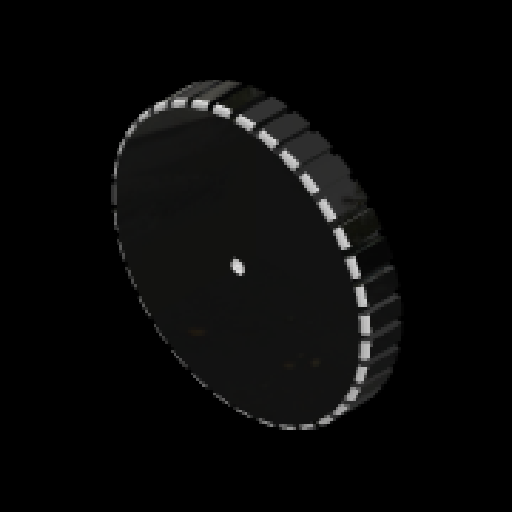
# Autodesk Inventor part: RobotWheelMK1
Saved by Autodesk Inventor 2025 (Build 290162000, 162)
## iProperties
Created: 2024-11-18
Part Number: RobotWheelMK1
Material: Generic
Document SubType Name: Modeling
Designer: Trevor
Density: 1 g/cm^3
Appearance: Default
Author: Trevor
Autodesk Inventor part; units mm, degrees
ref_plane "YZ Plane" through (0, 0, 0) normal (1, 0, 0) x (0, 1, 0)
ref_plane "XZ Plane" through (0, 0, 0) normal (0, 1, 0) x (-1, 0, 0)
sketch "Sketch1" plane through (0, 0, 0) normal (0, 0, 1) x (1, 0, 0)
  line L0 (-2.4408, -0.5408) -> (-1.2026, 2.1918) projected
  arc A0 (-2.4408, -0.5408) -> (-1.2026, 2.1918) centre (0, 0) ccw projected
  circle A1 centre (0, 0) radius 50
  line L1 (-52.2966, -3.2808) -> (-49.8922, -3.2808)
  line L2 (-49.8922, 3.2808) -> (-52.2966, 3.2808)
  line L3 (-52.2966, 3.2808) -> (-52.2966, -3.2808)
  line L4 (-52.2966, -3.2808) -> (-50, 0) construction
  line L5 (-50, 0) -> (-52.2966, 3.2808) construction
  line L6 (-49.6763, -5.6805) -> (-52.042, -6.1098)
  line L7 (-52.042, -6.1098) -> (-50.8703, -12.566)
  line L8 (-50.8703, -12.566) -> (-48.5046, -12.1367)
  circle A2 centre (0, 0) radius 50
  line L9 (-47.8637, -14.4592) -> (-50.1147, -15.3041)
  line L10 (-50.1147, -15.3041) -> (-47.8091, -21.4473)
  line L11 (-47.8091, -21.4473) -> (-45.5581, -20.6025)
  circle A3 centre (0, 0) radius 50
  line L12 (-44.5127, -22.7733) -> (-46.5767, -24.0064)
  line L13 (-46.5767, -24.0064) -> (-43.2112, -29.6393)
  line L14 (-43.2112, -29.6393) -> (-41.1472, -28.4061)
  circle A4 centre (0, 0) radius 50
  line L15 (-39.731, -30.3553) -> (-41.5417, -31.9372)
  line L16 (-41.5417, -31.9372) -> (-37.2245, -36.8787)
  line L17 (-37.2245, -36.8787) -> (-35.4138, -35.2967)
  circle A5 centre (0, 0) radius 50
  line L18 (-33.6724, -36.9618) -> (-35.1715, -38.8415)
  line L19 (-35.1715, -38.8415) -> (-30.0413, -42.9327)
  line L20 (-30.0413, -42.9327) -> (-28.5422, -41.0529)
  circle A6 centre (0, 0) radius 50
  line L21 (-26.5315, -42.3802) -> (-27.6708, -44.4975)
  line L22 (-27.6708, -44.4975) -> (-21.8926, -47.6068)
  line L23 (-21.8926, -47.6068) -> (-20.7533, -45.4896)
  circle A7 centre (0, 0) radius 50
  line L24 (-18.5378, -46.4365) -> (-19.2808, -48.7232)
  line L25 (-19.2808, -48.7232) -> (-13.0403, -50.7508)
  line L26 (-13.0403, -50.7508) -> (-12.2973, -48.4642)
  circle A8 centre (0, 0) radius 50
  line L27 (-9.9483, -49.0003) -> (-10.2711, -51.3829)
  line L28 (-10.2711, -51.3829) -> (-3.7688, -52.2637)
  line L29 (-3.7688, -52.2637) -> (-3.4461, -49.8811)
  circle A9 centre (0, 0) radius 50
  line L30 (-1.0391, -49.9892) -> (-0.9313, -52.3911)
  line L31 (-0.9313, -52.3911) -> (5.6238, -52.0967)
  line L32 (5.6238, -52.0967) -> (5.5159, -49.6948)
  circle A10 centre (0, 0) radius 50
  line L33 (7.9035, -49.3714) -> (8.4385, -51.7155)
  line L34 (8.4385, -51.7155) -> (14.8357, -50.2553)
  line L35 (14.8357, -50.2553) -> (14.3007, -47.9113)
  circle A11 centre (0, 0) radius 50
  line L36 (16.5921, -47.1668) -> (17.537, -49.3776)
  line L37 (17.537, -49.3776) -> (23.5707, -46.7987)
  line L38 (23.5707, -46.7987) -> (22.6257, -44.5879)
  circle A12 centre (0, 0) radius 50
  line L39 (24.7474, -43.4461) -> (26.0719, -45.4527)
  line L40 (26.0719, -45.4527) -> (31.5481, -41.8379)
  line L41 (31.5481, -41.8379) -> (30.2236, -39.8313)
  circle A13 centre (0, 0) radius 50
  line L42 (32.1073, -38.3291) -> (33.7688, -40.067)
  line L43 (33.7688, -40.067) -> (38.5116, -35.5324)
  line L44 (38.5116, -35.5324) -> (36.85, -33.7946)
  circle A14 centre (0, 0) radius 50
  line L45 (38.4352, -31.9802) -> (40.3804, -33.3934)
  line L46 (40.3804, -33.3934) -> (44.2373, -28.0849)
  line L47 (44.2373, -28.0849) -> (42.2921, -26.6717)
  circle A15 centre (0, 0) radius 50
  line L48 (43.5279, -24.6034) -> (45.6941, -25.6466)
  line L49 (45.6941, -25.6466) -> (48.5411, -19.7347)
  line L50 (48.5411, -19.7347) -> (46.3749, -18.6915)
  circle A16 centre (0, 0) radius 50
  line L51 (47.2214, -16.4358) -> (49.5391, -17.0754)
  line L52 (49.5391, -17.0754) -> (51.2848, -10.7502)
  line L53 (51.2848, -10.7502) -> (48.9671, -10.1106)
  circle A17 centre (0, 0) radius 50
  line L54 (49.3973, -7.7399) -> (51.792, -7.9555)
  line L55 (51.792, -7.9555) -> (52.3801, -1.4202)
  line L56 (52.3801, -1.4202) -> (49.9855, -1.2047)
  circle A18 centre (0, 0) radius 50
  line L57 (49.9855, 1.2047) -> (52.3801, 1.4202)
  line L58 (52.3801, 1.4202) -> (51.792, 7.9555)
  line L59 (51.792, 7.9555) -> (49.3973, 7.7399)
  circle A19 centre (0, 0) radius 50
  line L60 (48.9671, 10.1106) -> (51.2848, 10.7502)
  line L61 (51.2848, 10.7502) -> (49.5391, 17.0754)
  line L62 (49.5391, 17.0754) -> (47.2214, 16.4358)
  circle A20 centre (0, 0) radius 50
  line L63 (46.3749, 18.6915) -> (48.5411, 19.7347)
  line L64 (48.5411, 19.7347) -> (45.6941, 25.6466)
  line L65 (45.6941, 25.6466) -> (43.5279, 24.6034)
  circle A21 centre (0, 0) radius 50
  line L66 (42.2921, 26.6717) -> (44.2373, 28.0849)
  line L67 (44.2373, 28.0849) -> (40.3804, 33.3934)
  line L68 (40.3804, 33.3934) -> (38.4352, 31.9802)
  circle A22 centre (0, 0) radius 50
  line L69 (36.85, 33.7946) -> (38.5116, 35.5324)
  line L70 (38.5116, 35.5324) -> (33.7688, 40.067)
  line L71 (33.7688, 40.067) -> (32.1073, 38.3291)
  circle A23 centre (0, 0) radius 50
  line L72 (30.2236, 39.8313) -> (31.5481, 41.8379)
  line L73 (31.5481, 41.8379) -> (26.0719, 45.4527)
  line L74 (26.0719, 45.4527) -> (24.7474, 43.4461)
  circle A24 centre (0, 0) radius 50
  line L75 (22.6257, 44.5879) -> (23.5707, 46.7987)
  line L76 (23.5707, 46.7987) -> (17.537, 49.3776)
  line L77 (17.537, 49.3776) -> (16.5921, 47.1668)
  circle A25 centre (0, 0) radius 50
  line L78 (14.3007, 47.9113) -> (14.8357, 50.2553)
  line L79 (14.8357, 50.2553) -> (8.4385, 51.7155)
  line L80 (8.4385, 51.7155) -> (7.9035, 49.3714)
  circle A26 centre (0, 0) radius 50
  line L81 (5.5159, 49.6948) -> (5.6238, 52.0967)
  line L82 (5.6238, 52.0967) -> (-0.9313, 52.3911)
  line L83 (-0.9313, 52.3911) -> (-1.0391, 49.9892)
  circle A27 centre (0, 0) radius 50
  line L84 (-3.4461, 49.8811) -> (-3.7688, 52.2637)
  line L85 (-3.7688, 52.2637) -> (-10.2711, 51.3829)
  line L86 (-10.2711, 51.3829) -> (-9.9483, 49.0003)
  circle A28 centre (0, 0) radius 50
  line L87 (-12.2973, 48.4642) -> (-13.0403, 50.7508)
  line L88 (-13.0403, 50.7508) -> (-19.2808, 48.7232)
  line L89 (-19.2808, 48.7232) -> (-18.5378, 46.4365)
  circle A29 centre (0, 0) radius 50
  line L90 (-20.7533, 45.4896) -> (-21.8926, 47.6068)
  line L91 (-21.8926, 47.6068) -> (-27.6708, 44.4975)
  line L92 (-27.6708, 44.4975) -> (-26.5315, 42.3802)
  circle A30 centre (0, 0) radius 50
  line L93 (-28.5422, 41.0529) -> (-30.0413, 42.9327)
  line L94 (-30.0413, 42.9327) -> (-35.1715, 38.8415)
  line L95 (-35.1715, 38.8415) -> (-33.6724, 36.9618)
  circle A31 centre (0, 0) radius 50
  line L96 (-35.4138, 35.2967) -> (-37.2245, 36.8787)
  line L97 (-37.2245, 36.8787) -> (-41.5417, 31.9372)
  line L98 (-41.5417, 31.9372) -> (-39.731, 30.3553)
  circle A32 centre (0, 0) radius 50
  line L99 (-41.1472, 28.4061) -> (-43.2112, 29.6393)
  line L100 (-43.2112, 29.6393) -> (-46.5767, 24.0064)
  line L101 (-46.5767, 24.0064) -> (-44.5127, 22.7733)
  circle A33 centre (0, 0) radius 50
  line L102 (-45.5581, 20.6025) -> (-47.8091, 21.4473)
  line L103 (-47.8091, 21.4473) -> (-50.1147, 15.3041)
  line L104 (-50.1147, 15.3041) -> (-47.8637, 14.4592)
  circle A34 centre (0, 0) radius 50
  line L105 (-48.5046, 12.1367) -> (-50.8703, 12.566)
  line L106 (-50.8703, 12.566) -> (-52.042, 6.1098)
  line L107 (-52.042, 6.1098) -> (-49.6763, 5.6805)
  circle A35 centre (0, 0) radius 50
  line L108 (-1.3578, 2.3337) -> (-2.6499, -0.5177)
  arc A36 (-2.6499, -0.5177) -> (-1.3578, 2.3337) centre (0, 0) ccw
  point P0 (0, 0)
  point P1 (-49.1965, -8.9278)
  point P2 (-46.8117, -17.5687)
  point P3 (-42.9224, -25.645)
  point P4 (-37.6536, -32.8969)
  point P5 (-31.1745, -39.0916)
  point P6 (-23.6934, -44.0298)
  point P7 (-15.4508, -47.5528)
  point P8 (-6.7117, -49.5475)
  point P9 (2.2432, -49.9497)
  point P10 (11.126, -48.7464)
  point P11 (19.6513, -45.9764)
  point P12 (27.5448, -41.7287)
  point P13 (34.5531, -36.1397)
  point P14 (40.4508, -29.3893)
  point P15 (45.0484, -21.6942)
  point P16 (48.1981, -13.3018)
  point P17 (49.7987, -4.482)
  point P18 (49.7987, 4.482)
  point P19 (48.1981, 13.3018)
  point P20 (45.0484, 21.6942)
  point P21 (40.4508, 29.3893)
  point P22 (34.5531, 36.1397)
  point P23 (27.5448, 41.7287)
  point P24 (19.6513, 45.9764)
  point P25 (11.126, 48.7464)
  point P26 (2.2432, 49.9497)
  point P27 (-6.7117, 49.5475)
  point P28 (-15.4508, 47.5528)
  point P29 (-23.6934, 44.0298)
  point P30 (-31.1745, 39.0916)
  point P31 (-37.6536, 32.8969)
  point P32 (-42.9224, 25.645)
  point P33 (-46.8117, 17.5687)
  point P34 (-49.1965, 8.9278)
  dimension "d0" = 100
  dimension "d5" = 360
  dimension "d9" = 0.2
  constraints: 216 end point, 104 point on circle, 35 centre point, 2 coincident with centre, 1 coincident, 1 horizontal, 1 parallel, 355 other
  measures "d9" radial gap between concentric circles of A0 A36
ref_plane "Work Plane1" through (-2, -2, 15) normal (0, 0, 1) x (1, 0, 0)
extrude "Extrusion1" add sketch "Sketch1" along normal up to surface (15 mm away) contours A1 | A1 L59 L58 L57 | L56 L55 L54 A1 | A1 L62 L61 L60 | L53 L52 L51 A1 | A1 L65 L64 L63 | L50 L49 L48 A1 | A1 L68 L67 L66 | L47 L46 L45 A1 | A1 L71 L70 L69 | L44 L43 L42 A1 | A1 L74 L73 L72 | L41 L40 L39 A1 | A1 L77 L76 L75 | L38 L37 L36 A1 | A1 L80 L79 L78 | L35 L34 L33 A1 | A1 L83 L82 L81 | L32 L31 L30 A1 | A1 L86 L85 L84 | L29 L28 L27 A1 | A1 L89 L88 L87 | L26 L25 L24 A1 | A1 L92 L91 L90 | L23 L22 L21 A1 | A1 L95 L94 L93 | L20 L19 L18 A1 | A1 L98 L97 L96 | L17 L16 L15 A1 | A1 L101 L100 L99 | L14 L13 L12 A1 | A1 L104 L103 L102 | L11 L10 L9 A1 | A1 L107 L106 L105 | L8 L7 L6 A1 | A1 L1 L3 L2
fillet "Fillet1" radius 2 35 edges at (50.412, -13.9128, 15) (47.1176, -22.6906, 15) (42.3088, -30.7392, 15) (36.1402, -37.7997, 15) (28.81, -43.6453, 15) (20.5539, -48.0882, 15) (11.6371, -50.9854, 15) (2.3463, -52.2439, 15) (-7.0199, -51.8233, 15) (-16.1605, -49.737, 15) (-24.7817, -46.0521, 15) (-32.6064, -40.8871, 15) (-39.3831, -34.408, 15) (-44.8939, -26.8229, 15) (-48.9619, -18.3757, 15) (-51.4562, -9.3379, 15) (-52.2966, 0, 15) (-51.4562, 9.3379, 15) (-48.9619, 18.3757, 15) (-44.8939, 26.8229, 15) (-39.3831, 34.408, 15) (-32.6064, 40.8871, 15) (-24.7817, 46.0521, 15) (-16.1605, 49.737, 15) (-7.0199, 51.8233, 15) (2.3463, 52.2439, 15) (11.6371, 50.9854, 15) (20.5539, 48.0882, 15) (28.81, 43.6453, 15) (36.1402, 37.7997, 15) (42.3088, 30.7392, 15) (47.1176, 22.6906, 15) (50.412, 13.9128, 15) (52.0861, 4.6878, 15) (52.0861, -4.6878, 15)
fillet "Fillet2" radius 2 35 edges at (52.0861, 4.6878, 0) (50.412, 13.9128, 0) (47.1176, 22.6906, 0) (42.3088, 30.7392, 0) (36.1402, 37.7997, 0) (28.81, 43.6453, 0) (20.5539, 48.0882, 0) (11.6371, 50.9854, 0) (2.3463, 52.2439, 0) (-7.0199, 51.8233, 0) (-16.1605, 49.737, 0) (-24.7817, 46.0521, 0) (-32.6064, 40.8871, 0) (-39.3831, 34.408, 0) (-44.8939, 26.8229, 0) (-48.9619, 18.3757, 0) (-51.4562, 9.3379, 0) (-52.2966, 0, 0) (-51.4562, -9.3379, 0) (-48.9619, -18.3757, 0) (-44.8939, -26.8229, 0) (-39.3831, -34.408, 0) (-32.6064, -40.8871, 0) (-24.7817, -46.0521, 0) (-16.1605, -49.737, 0) (-7.0199, -51.8233, 0) (2.3463, -52.2439, 0) (11.6371, -50.9854, 0) (20.5539, -48.0882, 0) (28.81, -43.6453, 0) (36.1402, -37.7997, 0) (42.3088, -30.7392, 0) (47.1176, -22.6906, 0) (50.412, -13.9128, 0) (52.0861, -4.6878, 0)
fillet "Fillet3" radius 2 350 edges at (50.7201, 10.5944, 14.4142) (49.162, 10.1644, 15) (50.7201, 10.5944, 0.5858) (49.162, 10.1644, 0) (51.2848, 10.7502, 7.5) (48.9745, 16.9196, 14.4142) (47.4163, 16.4896, 15) (48.9745, 16.9196, 0.5858) (47.4163, 16.4896, 0) (49.5391, 17.0754, 7.5) (48.0133, 19.4805, 14.4142) (46.557, 18.7792, 15) (48.0133, 19.4805, 0.5858) (46.557, 18.7792, 0) (48.5411, 19.7347, 7.5) (45.1663, 25.3924, 14.4142) (43.71, 24.6911, 15) (45.1663, 25.3924, 0.5858) (43.71, 24.6911, 0) (45.6941, 25.6466, 7.5) (43.7633, 27.7406, 14.4142) (42.4557, 26.7905, 15) (43.7633, 27.7406, 0.5858) (42.4557, 26.7905, 0) (44.2373, 28.0849, 7.5) (40.3804, 33.3934, 7.5) (39.9065, 33.0491, 14.4142) (38.5988, 32.099, 15) (38.5988, 32.099, 0) (39.9065, 33.0491, 0.5858) (38.1068, 35.109, 14.4142) (36.9898, 33.9407, 15) (38.1068, 35.109, 0.5858) (36.9898, 33.9407, 0) (38.5116, 35.5324, 7.5) (33.7688, 40.067, 7.5) (33.364, 39.6436, 14.4142) (32.247, 38.4753, 15) (32.247, 38.4753, 0) (33.364, 39.6436, 0.5858) (30.335, 40.0001, 0) (31.5481, 41.8379, 7.5) (31.2254, 41.349, 14.4142) (30.335, 40.0001, 15) (31.2254, 41.349, 0.5858) (26.0719, 45.4527, 7.5) (25.7492, 44.9639, 14.4142) (24.8588, 43.6149, 15) (24.8588, 43.6149, 0) (25.7492, 44.9639, 0.5858) (22.7052, 44.7738, 0) (23.5707, 46.7987, 7.5) (23.3405, 46.2601, 14.4142) (22.7052, 44.7738, 15) (23.3405, 46.2601, 0.5858) (17.537, 49.3776, 7.5) (17.3068, 48.839, 14.4142) (16.6715, 47.3527, 15) (16.6715, 47.3527, 0) (17.3068, 48.839, 0.5858) (14.7053, 49.6842, 14.4142) (14.3456, 48.1084, 15) (14.7053, 49.6842, 0.5858) (14.3456, 48.1084, 0) (14.8357, 50.2553, 7.5) (8.3082, 51.1444, 14.4142) (7.9485, 49.5685, 15) (8.3082, 51.1444, 0.5858) (7.9485, 49.5685, 0) (8.4385, 51.7155, 7.5) (-0.9575, 51.8059, 14.4142) (-1.0301, 50.1912, 15) (-0.9575, 51.8059, 0.5858) (-1.0301, 50.1912, 0) (-0.9313, 52.3911, 7.5) (5.5975, 51.5115, 14.4142) (5.525, 49.8968, 15) (5.5975, 51.5115, 0.5858) (5.525, 49.8968, 0) (5.6238, 52.0967, 7.5) (-3.6902, 51.6832, 14.4142) (-3.4732, 50.0814, 15) (-3.6902, 51.6832, 0.5858) (-3.4732, 50.0814, 0) (-3.7688, 52.2637, 7.5) (-10.1925, 50.8024, 14.4142) (-9.9755, 49.2007, 15) (-10.1925, 50.8024, 0.5858) (-9.9755, 49.2007, 0) (-10.2711, 51.3829, 7.5) (-12.8593, 50.1937, 14.4142) (-12.3598, 48.6565, 15) (-12.8593, 50.1937, 0.5858) (-12.3598, 48.6565, 0) (-13.0403, 50.7508, 7.5) (-19.0998, 48.1661, 14.4142) (-18.6003, 46.6288, 15) (-19.0998, 48.1661, 0.5858) (-18.6003, 46.6288, 0) (-19.2808, 48.7232, 7.5) (-21.615, 47.091, 14.4142) (-20.8491, 45.6676, 15) (-21.615, 47.091, 0.5858) (-20.8491, 45.6676, 0) (-21.8926, 47.6068, 7.5) (-27.3932, 43.9816, 14.4142) (-26.6273, 42.5582, 15) (-27.3932, 43.9816, 0.5858) (-26.6273, 42.5582, 0) (-27.6708, 44.4975, 7.5) (-29.6761, 42.4747, 14.4142) (-28.6683, 41.211, 15) (-29.6761, 42.4747, 0.5858) (-28.6683, 41.211, 0) (-30.0413, 42.9327, 7.5) (-34.8062, 38.3836, 14.4142) (-33.7984, 37.1198, 15) (-34.8062, 38.3836, 0.5858) (-33.7984, 37.1198, 0) (-35.1715, 38.8415, 7.5) (-36.7833, 36.4932, 14.4142) (-35.5661, 35.4298, 15) (-36.7833, 36.4932, 0.5858) (-35.5661, 35.4298, 0) (-37.2245, 36.8787, 7.5) (-41.1005, 31.5518, 14.4142) (-39.8833, 30.4883, 15) (-41.1005, 31.5518, 0.5858) (-39.8833, 30.4883, 0) (-41.5417, 31.9372, 7.5) (-46.0738, 23.706, 14.4142) (-44.6862, 22.877, 15) (-46.0738, 23.706, 0.5858) (-44.6862, 22.877, 0) (-46.5767, 24.0064, 7.5) (-42.7083, 29.3389, 14.4142) (-41.3208, 28.5098, 15) (-42.7083, 29.3389, 0.5858) (-41.3208, 28.5098, 0) (-43.2112, 29.6393, 7.5) (-47.2607, 21.2415, 14.4142) (-45.7473, 20.6736, 15) (-47.2607, 21.2415, 0.5858) (-45.7473, 20.6736, 0) (-47.8091, 21.4473, 7.5) (-49.5663, 15.0982, 14.4142) (-48.0529, 14.5303, 15) (-49.5663, 15.0982, 0.5858) (-48.0529, 14.5303, 0) (-50.1147, 15.3041, 7.5) (-50.294, 12.4614, 14.4142) (-48.7036, 12.1728, 15) (-50.294, 12.4614, 0.5858) (-48.7036, 12.1728, 0) (-50.8703, 12.566, 7.5) (-51.4656, 6.0052, 14.4142) (-49.8752, 5.7166, 15) (-51.4656, 6.0052, 0.5858) (-49.8752, 5.7166, 0) (-52.042, 6.1098, 7.5) (-51.7108, 3.2808, 14.4142) (-50.0944, 3.2808, 15) (-51.7108, 3.2808, 0.5858) (-50.0944, 3.2808, 0) (-52.2966, 3.2808, 7.5) (-51.7108, -3.2808, 14.4142) (-50.0944, -3.2808, 15) (-51.7108, -3.2808, 0.5858) (-50.0944, -3.2808, 0) (-52.2966, -3.2808, 7.5) (51.7967, 1.3677, 14.4142) (50.1868, 1.2228, 15) (51.7967, 1.3677, 0.5858) (50.1868, 1.2228, 0) (52.3801, 1.4202, 7.5) (51.2085, 7.903, 14.4142) (49.5987, 7.7581, 15) (51.2085, 7.903, 0.5858) (49.5987, 7.7581, 0) (51.792, 7.9555, 7.5) (51.7967, -1.3677, 14.4142) (50.1868, -1.2228, 15) (51.7967, -1.3677, 0.5858) (50.1868, -1.2228, 0) (52.3801, -1.4202, 7.5) (51.2085, -7.903, 14.4142) (49.5987, -7.7581, 15) (51.2085, -7.903, 0.5858) (49.5987, -7.7581, 0) (51.792, -7.9555, 7.5) (48.9745, -16.9196, 14.4142) (47.4163, -16.4896, 15) (48.9745, -16.9196, 0.5858) (47.4163, -16.4896, 0) (49.5391, -17.0754, 7.5) (50.7201, -10.5944, 14.4142) (49.162, -10.1644, 15) (50.7201, -10.5944, 0.5858) (49.162, -10.1644, 0) (51.2848, -10.7502, 7.5) (48.0133, -19.4805, 14.4142) (46.557, -18.7792, 15) (48.0133, -19.4805, 0.5858) (46.557, -18.7792, 0) (48.5411, -19.7347, 7.5) (45.1663, -25.3924, 14.4142) (43.71, -24.6911, 15) (45.1663, -25.3924, 0.5858) (43.71, -24.6911, 0) (45.6941, -25.6466, 7.5) (43.7633, -27.7406, 14.4142) (42.4557, -26.7905, 15) (43.7633, -27.7406, 0.5858) (42.4557, -26.7905, 0) (44.2373, -28.0849, 7.5) (39.9065, -33.0491, 14.4142) (38.5988, -32.099, 15) (39.9065, -33.0491, 0.5858) (38.5988, -32.099, 0) (40.3804, -33.3934, 7.5) (38.1068, -35.109, 14.4142) (36.9898, -33.9407, 15) (38.1068, -35.109, 0.5858) (36.9898, -33.9407, 0) (38.5116, -35.5324, 7.5) (33.364, -39.6436, 14.4142) (32.247, -38.4753, 15) (33.364, -39.6436, 0.5858) (32.247, -38.4753, 0) (33.7688, -40.067, 7.5) (25.7492, -44.9639, 14.4142) (24.8588, -43.6149, 15) (25.7492, -44.9639, 0.5858) (24.8588, -43.6149, 0) (26.0719, -45.4527, 7.5) (31.2254, -41.349, 14.4142) (30.335, -40.0001, 15) (31.2254, -41.349, 0.5858) (30.335, -40.0001, 0) (31.5481, -41.8379, 7.5) (23.3405, -46.2601, 14.4142) (22.7052, -44.7738, 15) (23.3405, -46.2601, 0.5858) (22.7052, -44.7738, 0) (23.5707, -46.7987, 7.5) (17.3068, -48.839, 14.4142) (16.6715, -47.3527, 15) (17.3068, -48.839, 0.5858) (16.6715, -47.3527, 0) (17.537, -49.3776, 7.5) (14.7053, -49.6842, 14.4142) (14.3456, -48.1084, 15) (14.7053, -49.6842, 0.5858) (14.3456, -48.1084, 0) (14.8357, -50.2553, 7.5) (8.3082, -51.1444, 14.4142) (7.9485, -49.5685, 15) (8.3082, -51.1444, 0.5858) (7.9485, -49.5685, 0) (8.4385, -51.7155, 7.5) (5.5975, -51.5115, 14.4142) (5.525, -49.8968, 15) (5.5975, -51.5115, 0.5858) (5.525, -49.8968, 0) (5.6238, -52.0967, 7.5) (-3.6902, -51.6832, 14.4142) (-3.4732, -50.0814, 15) (-3.6902, -51.6832, 0.5858) (-3.4732, -50.0814, 0) (-3.7688, -52.2637, 7.5) (-10.1925, -50.8024, 14.4142) (-9.9755, -49.2007, 15) (-10.1925, -50.8024, 0.5858) (-9.9755, -49.2007, 0) (-10.2711, -51.3829, 7.5) (-50.294, -12.4614, 14.4142) (-48.7036, -12.1728, 15) (-50.294, -12.4614, 0.5858) (-48.7036, -12.1728, 0) (-50.8703, -12.566, 7.5) (-47.2607, -21.2415, 14.4142) (-45.7473, -20.6736, 15) (-47.2607, -21.2415, 0.5858) (-45.7473, -20.6736, 0) (-47.8091, -21.4473, 7.5) (-42.7083, -29.3389, 14.4142) (-41.3208, -28.5098, 15) (-42.7083, -29.3389, 0.5858) (-41.3208, -28.5098, 0) (-43.2112, -29.6393, 7.5) (-36.7833, -36.4932, 14.4142) (-35.5661, -35.4298, 15) (-36.7833, -36.4932, 0.5858) (-35.5661, -35.4298, 0) (-37.2245, -36.8787, 7.5) (-29.6761, -42.4747, 14.4142) (-28.6683, -41.211, 15) (-29.6761, -42.4747, 0.5858) (-28.6683, -41.211, 0) (-30.0413, -42.9327, 7.5) (-21.615, -47.091, 14.4142) (-20.8491, -45.6676, 15) (-21.615, -47.091, 0.5858) (-20.8491, -45.6676, 0) (-21.8926, -47.6068, 7.5) (-12.8593, -50.1937, 14.4142) (-12.3598, -48.6565, 15) (-12.8593, -50.1937, 0.5858) (-12.3598, -48.6565, 0) (-13.0403, -50.7508, 7.5) (-19.0998, -48.1661, 14.4142) (-18.6003, -46.6288, 15) (-19.0998, -48.1661, 0.5858) (-18.6003, -46.6288, 0) (-19.2808, -48.7232, 7.5) (-27.3932, -43.9816, 14.4142) (-26.6273, -42.5582, 15) (-27.3932, -43.9816, 0.5858) (-26.6273, -42.5582, 0) (-27.6708, -44.4975, 7.5) (-34.8062, -38.3836, 14.4142) (-33.7984, -37.1198, 15) (-34.8062, -38.3836, 0.5858) (-33.7984, -37.1198, 0) (-35.1715, -38.8415, 7.5) (-41.1005, -31.5518, 14.4142) (-39.8833, -30.4883, 15) (-41.1005, -31.5518, 0.5858) (-39.8833, -30.4883, 0) (-41.5417, -31.9372, 7.5) (-46.0738, -23.706, 14.4142) (-44.6862, -22.877, 15) (-46.0738, -23.706, 0.5858) (-44.6862, -22.877, 0) (-46.5767, -24.0064, 7.5) (-49.5663, -15.0982, 14.4142) (-48.0529, -14.5303, 15) (-49.5663, -15.0982, 0.5858) (-48.0529, -14.5303, 0) (-50.1147, -15.3041, 7.5) (-51.4656, -6.0052, 14.4142) (-49.8752, -5.7166, 15) (-51.4656, -6.0052, 0.5858) (-49.8752, -5.7166, 0) (-52.042, -6.1098, 7.5) (-0.9575, -51.8059, 14.4142) (-1.0301, -50.1912, 15) (-0.9575, -51.8059, 0.5858) (-1.0301, -50.1912, 0) (-0.9313, -52.3911, 7.5)
body "Solid1"
